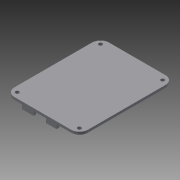
# Autodesk Inventor part: obudowa - budzik v3 dol dol
Saved by Autodesk Inventor 2014 (Build 180170000, 170)
## iProperties
Created: 2018-03-05
Part Number: obudowa - budzik v3 dol dol
Material: Generic
Document SubType Name: Modeling
Designer: HP820
Density: 1 g/cm^3
Appearance: Default
Author: HP820
Autodesk Inventor part; units mm, degrees
ref_plane "YZ Plane" through (0, 0, 0) normal (1, 0, 0) x (0, 1, 0)
ref_plane "XZ Plane" through (0, 0, 0) normal (0, 1, 0) x (-1, 0, 0)
ref_plane "XY Plane" through (0, 0, 0) normal (0, 0, 1) x (1, 0, 0)
sketch "Sketch1" plane through (0, 0, 0) normal (0, 0, 1) x (1, 0, 0)
  circle A0 centre (29.5808, -39.6651) radius 1.75 projected
  circle A1 centre (-29.5808, 39.6651) radius 1.75 projected
  circle A2 centre (29.5808, 39.6651) radius 1.75 projected
  circle A3 centre (-29.5808, -39.6651) radius 1.75 projected
  line L0 (13.1764, -42.5) -> (13.1764, -45) projected
  line L1 (13.1764, -45) -> (27, -45) projected
  arc A4 (27, -45) -> (35, -37) centre (27, -37) ccw projected
  line L2 (35, -37) -> (35, 36.8048) projected
  ellipse E0 centre (27, 36.8048) end of major axis (27, 45) minor radius 8 (35, 36.8048) -> (27, 45) ccw projected
  line L3 (27, 45) -> (-27, 45) projected
  ellipse E1 centre (-27, 36.8048) end of major axis (-27, 45) minor radius 8 (-27, 45) -> (-35, 36.8048) ccw projected
  line L4 (-35, 36.8048) -> (-35, -37) projected
  arc A5 (-35, -37) -> (-27, -45) centre (-27, -37) ccw projected
  line L5 (-27, -45) -> (-19.7694, -45) projected
  line L6 (-19.7694, -45) -> (-19.7694, -42.5) projected
  line L7 (-19.7694, -42.5) -> (-22.5, -42.5) projected
  arc A6 (-24.2843, -42.3395) -> (-22.5, -42.5) centre (-22.5, -32.5) ccw projected
  arc A7 (-24.2843, -42.3395) -> (-32.4877, -32.9952) centre (-33.2764, -41.9606) ccw projected
  arc A8 (-32.5, -32.5) -> (-32.4877, -32.9952) centre (-22.5, -32.5) ccw projected
  line L8 (-32.5, -32.5) -> (-32.5, 32.2561) projected
  ellipse E2 centre (-22.5, 32.2561) end of major axis (-22.5, 42.5) minor radius 10 (-32.4132, 33.603) -> (-32.5, 32.2561) ccw projected
  arc A9 (-32.4132, 33.603) -> (-23.6584, 42.431) centre (-32.6569, 42.5997) ccw projected
  ellipse E3 centre (-22.5, 32.2561) end of major axis (-22.5, 42.5) minor radius 10 (-22.5, 42.5) -> (-23.6584, 42.431) ccw projected
  line L9 (-22.5, 42.5) -> (22.5, 42.5) projected
  ellipse E4 centre (22.5, 32.2561) end of major axis (22.5, 42.5) minor radius 10 (23.6584, 42.431) -> (22.5, 42.5) ccw projected
  arc A10 (23.6584, 42.431) -> (32.4132, 33.603) centre (32.6569, 42.5997) ccw projected
  ellipse E5 centre (22.5, 32.2561) end of major axis (22.5, 42.5) minor radius 10 (32.5, 32.2561) -> (32.4132, 33.603) ccw projected
  line L10 (32.5, 32.2561) -> (32.5, -32.5) projected
  arc A11 (32.4877, -32.9952) -> (32.5, -32.5) centre (22.5, -32.5) ccw projected
  arc A12 (32.4877, -32.9952) -> (24.2843, -42.3395) centre (33.2764, -41.9606) ccw projected
  arc A13 (22.5, -42.5) -> (24.2843, -42.3395) centre (22.5, -32.5) ccw projected
  line L11 (22.5, -42.5) -> (13.1764, -42.5) projected
  line L12 (-19.7694, -45) -> (13.1764, -45)
  point P0 (0, 0)
  constraints: 2 end point, 1 collinear, 6 other
extrude "Extrusion1" add sketch "Sketch1" along normal blind 2.4
sketch "Sketch2" plane through (0, 0, 0) normal (0, 0, -1) x (-1, 0, 0)
  line L0 (27, -45) -> (-27, -45) projected
  line L1 (-25, -35) -> (25, -35)
  line L2 (25, -35) -> (25, 25)
  line L3 (25, 25) -> (-25, 25)
  line L4 (-25, 25) -> (-25, -35)
  line L5 (-25, -35) -> (25, 25) construction
  line L6 (25, -35) -> (-25, 25) construction
  circle A0 centre (-25, 25) radius 1.25
  circle A1 centre (-25, 25) radius 3
  circle A2 centre (25, 25) radius 1.25
  circle A3 centre (25, 25) radius 3
  circle A4 centre (25, -35) radius 1.25
  circle A5 centre (25, -35) radius 3
  circle A6 centre (-25, -35) radius 1.25
  circle A7 centre (-25, -35) radius 3
  point P0 (0, 0)
  point P1 (0, -5)
  dimension "d2" = 50
  dimension "d3" = 60
  dimension "d4" = 10
  dimension "d5" = 2.5
  dimension "d6" = 6
  dimension "d7" = 2.5
  dimension "d8" = 6
  dimension "d9" = 2.5
  dimension "d10" = 6
  dimension "d11" = 2.5
  dimension "d12" = 6
  constraints: 12 end point, 8 centre point, 5 coincident, 2 midpoint, 2 parallel, 1 horizontal, 1 perpendicular
  measures "d2" distance of L3.end L2.end
  measures "d3" distance of L2.end L1.end
  measures "d4" distance between parallel lines of L0 L1
  measures "d5" diameter of A0
  measures "d6" diameter of A1
  measures "d7" diameter of A2
  measures "d8" diameter of A3
  measures "d9" diameter of A4
  measures "d10" diameter of A5
  measures "d11" diameter of A6
  measures "d12" diameter of A7
extrude "Extrusion2" add sketch "Sketch2" along normal blind 4 contours A6 L4 A7 L1 | L1 A7 L4 A6 | A5 L2 A4 L1 | L1 A4 L2 A5 | A1 L3 A0 L4 | L4 A0 L3 A1 | A3 L3 A2 L2 | L2 A2 L3 A3
sketch "Sketch3" plane through (0, 0, 0) normal (0, 0, -1) x (-1, 0, 0)
  line L0 (27, -45) -> (-27, -45) projected
  line L1 (-13.1764, -45) -> (-3.1764, -45) projected
  line L2 (8.7694, -45) -> (19.7694, -45) projected
  line L3 (-3.1764, -42.5) -> (-13.1764, -42.5) projected
  line L4 (-3.1764, -45) -> (-3.1764, -42.5) projected
  line L5 (-13.1764, -45) -> (-3.1764, -45) projected
  line L6 (-13.1764, -45) -> (-13.1764, -42.5) projected
  line L7 (19.7694, -42.5) -> (8.7694, -42.5) projected
  line L8 (19.7694, -45) -> (19.7694, -42.5) projected
  line L9 (8.7694, -45) -> (19.7694, -45) projected
  line L10 (8.7694, -45) -> (8.7694, -42.5) projected
  point P0 (0, 0)
extrude "Extrusion3" add sketch "Sketch3" along normal blind 4
body "Solid1"
